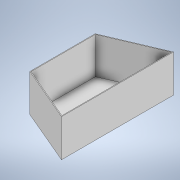
# Autodesk Inventor part: footprint
Saved by Autodesk Inventor 2021 (Build 250183000, 183)
## iProperties
Created: 2020-11-23
Part Number: footprint
Material: Generic
Document SubType Name: Modeling
Designer: gurle
Density: 1 g/cm^3
Appearance: Default
Author: gurle
Autodesk Inventor part; units mm, degrees
ref_plane "YZ Plane" through (0, 0, 0) normal (1, 0, 0) x (0, 1, 0)
ref_plane "XZ Plane" through (0, 0, 0) normal (0, 1, 0) x (-1, 0, 0)
ref_plane "XY Plane" through (0, 0, 0) normal (0, 0, 1) x (1, 0, 0)
sketch "Sketch1" plane through (0, 0, 0) normal (0, 1, 0) x (-1, 0, 0)
  line L0 (0, 0) -> (0, -152.4)
  line L1 (0, -152.4) -> (74.791, -120.6531)
  line L2 (74.791, -120.6531) -> (74.791, -31.7531)
  line L3 (74.791, -31.7531) -> (0, 0)
  dimension "d5" = 152.4
  dimension "d6" = 81.25
  dimension "d7" = 67
  dimension "d8" = 88.9
  constraints: 8 end point, 1 parallel, 1 vertical
  measures "d5" distance of L0.start L0.end
  measures "d6" distance of L0.end L1.end
  measures "d7" angle of L1 L0
  measures "d8" distance of L1.end L2.end
extrude "Extrusion1" add sketch "Sketch1" along normal blind 50.8
shell "Shell1" thickness 1 removed faces 1 at (-24.9303, 50.8, -61.3844)
body "Solid1"
